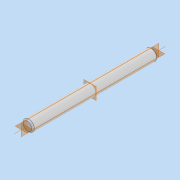
# Autodesk Inventor part: shaft4x45
Saved by Autodesk Inventor 2022 (Build 260153000, 153)
## iProperties
Created: 2024-04-23
Part Number: shaft4x45
Material: Generic
Document SubType Name: Modeling
Designer: ktamu
Density: 1 g/cm^3
Appearance: Default
Author: ktamu
Autodesk Inventor part; units mm, degrees
sketch "スケッチ1" plane through (0, 0, 0) normal (0, 0, 1) x (1, 0, 0)
  circle A0 centre (0, 0) radius 2
  dimension "d0" = 4
  constraints: 1 centre point, 1 coincident
  measures "d0" diameter of A0
extrude "押し出し1" add sketch "スケッチ1" along normal mid plane 45
chamfer "面取り1" distance 0.5 angle 45 1 edges at (-2, 0, 22.5)
chamfer "面取り2" distance 0.5 angle 45 1 edges at (-2, 0, -22.5)
